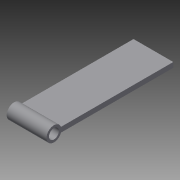
# Autodesk Inventor part: aimingrails
Saved by Autodesk Inventor 2016 (Build 200138000, 138)
## iProperties
Created: 2016-01-30
Part Number: aimingrails
Material: Generic
Document SubType Name: Modeling
Designer: zachary
Density: 1 g/cm^3
Appearance: Default
Author: zachary
Autodesk Inventor part; units mm, degrees
ref_plane "YZ Plane" through (0, 0, 0) normal (1, 0, 0) x (0, 1, 0)
ref_plane "XZ Plane" through (0, 0, 0) normal (0, 1, 0) x (-1, 0, 0)
ref_plane "XY Plane" through (0, 0, 0) normal (0, 0, 1) x (1, 0, 0)
sketch "Sketch1" plane through (0, 0, 0) normal (1, 0, 0) x (0, 1, 0)
  line L0 (3.175, -4.4901) -> (3.175, -71.7099)
  line L1 (0, -71.7099) -> (0, -4.4901)
  arc A0 (3.175, -4.4901) -> (0, -4.4901) centre (1.5875, 0) ccw
  circle A1 centre (1.5875, 0) radius 3.175
  circle A2 centre (1.5875, -76.2) radius 3.175
  arc A3 (0, -71.7099) -> (3.175, -71.7099) centre (1.5875, -76.2) ccw
  point P0 (0, 0)
  point P1 (0, -73.4504)
  dimension "d7" = 6.35
  dimension "d0" = 3.175
  dimension "d2" = 6.35
  dimension "d3" = 1.5875
  dimension "d6" = 1.5875
  constraints: 4 end point, 4 point on circle, 3 centre point, 2 coincident, 1 parallel, 3 other
  measures "d0" distance between parallel lines of L1 L0
  measures "d2" diameter of A1
  measures "d3" radial gap between concentric circles of A1 A0
extrude "Extrusion1" add sketch "Sketch1" along normal blind 25.4 contours L0 A3 L1 A0 | A2
sketch "Sketch2" plane through (25.4, 0, 0) normal (1, 0, 0) x (0, 0, -1)
  circle A0 centre (76.4423, 1.5875) radius 3.175
  arc A1 (71.7099, 0) -> (71.7099, 3.175) centre (76.2, 1.5875) ccw projected
  point P0 (0, 0)
  dimension "d8" = 0
  dimension "d9" = 6.35
  constraints: 1 centre point
  measures "d8" vertical distance of A0.centre A1.centre
  measures "d9" diameter of A0
extrude "Extrusion2" cut sketch "Sketch2" against normal through all
body "Solid1"
